Autodesk Inventor part; units mm, degrees
(part 2 of 2)
sketch "스케치56" plane through (122.9382, 45, 39.8809) normal (0.2220643, 0.975032, 0) x (0.975032, -0.2220643, 0)
  line L0 (18.3862, 42.8792) -> (34.3862, 42.8792)
  line L1 (34.3862, 42.8792) -> (34.3862, 36.8792)
  line L2 (34.3862, 36.8792) -> (18.3862, 36.8792)
  line L3 (18.3862, 36.8792) -> (18.3862, 42.8792)
  ellipse E0 centre (70.8617, 39.8792) end of major axis (70.8617, 31.8792) minor radius 7.8003 (74.099, 32.6007) -> (74.0934, 47.1603) ccw construction
  line L4 (70.8617, 39.8792) -> (98.8251, 39.8792) construction
  line L5 (18.3862, 39.8792) -> (34.3862, 39.8792) construction
  point P0 (-109.8758, 39.8809)
  dimension "d238" = 16
  dimension "d239" = 6
  dimension "d240" = 0
  constraints: 12 end point, 2 horizontal, 2 midpoint, 2 parallel, 1 perpendicular, 1 other
  measures "d238" distance of L1.end L2.end
  measures "d239" distance of L0.end L1.end
  measures "d240" distance from line of L4.start L5
extrude "돌출36" cut sketch "스케치56" against normal blind 22
